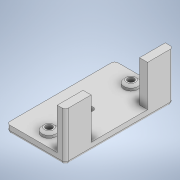
# Autodesk Inventor part: bigSpringBedMount
Saved by Autodesk Inventor 2022 (Build 260153000, 153)
## iProperties
Created: 2020-07-26
Part Number: bigSpringBedMount
Material: Generic
Document SubType Name: Modeling
Designer: PAB
Density: 1 g/cm^3
Appearance: Default
Author: PAB
Autodesk Inventor part; units mm, degrees
ref_plane "YZ Plane" through (0, 0, 0) normal (1, 0, 0) x (0, 1, 0)
ref_plane "XZ Plane" through (0, 0, 0) normal (0, 1, 0) x (-1, 0, 0)
ref_plane "XY Plane" through (0, 0, 0) normal (0, 0, 1) x (1, 0, 0)
sketch "Sketch1" plane through (0, 0, 0) normal (0, 1, 0) x (-1, 0, 0)
  line L0 (18.7, 33.5) -> (-17.7, 33.5)
  line L1 (-17.7, 33.5) -> (-17.7, -33.5)
  line L2 (-17.7, -33.5) -> (18.7, -33.5)
  line L3 (18.7, -33.5) -> (18.7, 33.5)
  point P0 (0, 0)
  dimension "d0" = 36.4
  dimension "d1" = 67
  constraints: 8 end point, 2 parallel, 1 horizontal, 1 perpendicular
  measures "d0" distance of L2.end L1.end
  measures "d1" distance of L1.end L0.end
extrude "Extrusion1" add sketch "Sketch1" along normal blind 5
sketch "Sketch2" plane through (0, 5, 0) normal (0, 1, 0) x (1, 0, 0)
  line L0 (-18.7, -33.5) -> (17.7, -33.5) projected
  line L1 (17.7, -33.5) -> (12.7, -33.5)
  line L2 (12.7, -33.5) -> (12.7, -12.5)
  line L3 (12.7, -12.5) -> (17.7, -12.5)
  line L4 (17.7, -12.5) -> (17.7, -33.5)
  line L5 (17.7, -33.5) -> (17.7, 33.5) projected
  line L6 (17.7, 33.5) -> (12.7, 33.5)
  line L7 (12.7, 33.5) -> (12.7, 12.5)
  line L8 (12.7, 12.5) -> (17.7, 12.5)
  line L9 (17.7, 12.5) -> (17.7, 33.5)
  point P0 (0, 0)
  dimension "d4" = 5
  dimension "d5" = 21
  dimension "d6" = 5
  dimension "d7" = 21
  constraints: 16 end point, 4 parallel, 2 horizontal, 2 perpendicular
  measures "d4" distance of L2.end L3.end
  measures "d5" distance of L1.end L2.end
  measures "d6" distance of L8.end L7.end
  measures "d7" distance of L7.end L6.end
extrude "Extrusion2" add sketch "Sketch2" along normal blind 25.4
fillet "Fillet2" radius 2 6 edges at (-0.5, 0, 33.5) (-18.7, 0, 0) (17.7, 15.2, 33.5) (17.7, 15.2, -33.5) (-0.5, 0, -33.5) (17.7, 0, 0)
sketch "Sketch6" plane through (0, 5, 0) normal (0, 1, 0) x (1, 0, 0)
  line L0 (-18.7, -33.5) -> (-18.7, 33.5) projected
  line L1 (-18.7, 12) -> (-13.7, 12)
  line L2 (-13.7, 12) -> (-13.7, -12)
  line L3 (-13.7, -12) -> (-18.7, -12)
  line L4 (-18.7, -12) -> (-18.7, 12)
  point P0 (0, 0)
  point P1 (-18.7, -12)
  dimension "d26" = 5
  dimension "d27" = 24
  constraints: 8 end point, 2 parallel, 1 horizontal, 1 perpendicular, 1 point on line
  measures "d26" distance of L2.end L3.end
  measures "d27" distance of L1.end L2.end
extrude "Extrusion6" add sketch "Sketch6" along normal blind 25.4
fillet "Fillet3" radius 2 4 edges at (-18.1142, 0.5858, 32.9142) (-18.7, 3.5, 33.5) (-18.1142, 0.5858, -32.9142) (-18.7, 3.5, -33.5)
sketch "Sketch8" plane through (0, 5, 0) normal (0, 1, 0) x (1, 0, 0)
  circle A0 centre (-0.5, 0) radius 4.325
  circle A1 centre (-0.5, -25.4) radius 4.325
  circle A2 centre (-0.5, 25.4) radius 4.325
  point P0 (0, 0)
  dimension "d37" = 8.65
  dimension "d38" = 8.65
  dimension "d39" = 8.65
  constraints: 3 centre point
  measures "d37" diameter of A0
  measures "d38" diameter of A1
  measures "d39" diameter of A2
extrude "Extrusion8" add sketch "Sketch8" along normal blind 3 contours A1 | A2
chamfer "Chamfer1" distance 1.5 angle 45 2 edges at (-4.825, 8, -25.4) (-4.825, 8, 25.4)
sketch "Sketch9" plane through (-0.5, 8, 0) normal (0, 1, 0) x (1, 0, 0)
  circle A0 centre (0, 0) radius 2.825 projected
  circle A1 centre (0, 0) radius 2
  circle A2 centre (0, 25.4) radius 2.825 projected
  circle A3 centre (0, 25.4) radius 2
  circle A4 centre (0, -25.4) radius 2.825 projected
  circle A5 centre (0, -25.4) radius 2
  point P0 (0.5, 0)
  dimension "d45" = 4
  dimension "d46" = 4
  dimension "d47" = 4
  constraints: 3 centre point, 3 coincident
  measures "d45" diameter of A1
  measures "d46" diameter of A3
  measures "d47" diameter of A5
extrude "Extrusion9" cut sketch "Sketch9" against normal blind 20 contours A1 | A3 | A5
sketch "Sketch10" plane through (0, 0, 0) normal (0, -1, 0) x (1, 0, 0)
  circle A0 centre (-0.5, -25.4) radius 2.825 projected
  circle A1 centre (-0.5, -25.4) radius 3
  circle A2 centre (-0.5, 0) radius 4.325 projected
  circle A3 centre (-0.5, 0) radius 3
  circle A4 centre (-0.5, 25.4) radius 2.825 projected
  circle A5 centre (-0.5, 25.4) radius 3
  point P0 (0, 0)
  dimension "d50" = 6
  dimension "d51" = 6
  dimension "d52" = 6
  constraints: 3 centre point, 3 coincident
  measures "d50" diameter of A1
  measures "d51" diameter of A3
  measures "d52" diameter of A5
extrude "Extrusion10" cut sketch "Sketch10" against normal blind 2.5 contours A0 | A1 | A4 | A5
sketch "Sketch11" plane through (-18.7, 5, 12) normal (-1, 0, 0) x (0, 0, 1)
  line L0 (21.5, 0) -> (0.5, 0) projected
  line L1 (-29.5, 29.5575) -> (5.5, 29.5575)
  line L2 (5.5, 29.5575) -> (5.5, 0)
  line L3 (5.5, 0) -> (-29.5, 0)
  line L4 (-29.5, 0) -> (-29.5, 29.5575)
  point P0 (-12, -5)
  dimension "d55" = 35
  constraints: 8 end point, 2 parallel, 1 horizontal, 1 perpendicular, 1 point on line
  measures "d55" distance of L2.end L3.end
extrude "Extrusion11" cut sketch "Sketch11" against normal blind 50
body "Solid1"
